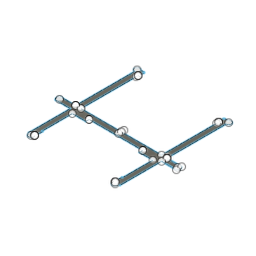
4~6F廊下用平面[少し幅大きく作ったから修正入れていこう] (Autodesk Fusion 360 design; units mm, degrees)
Autodesk Fusion 360 part; units mm, degrees
sketch "スケッチ1" plane through (0, 0, 0) normal (0, 0, 1) x (1, 0, 0)
  line L0 (-14000, -4000) -> (-54000, -4000)
  line L1 (-4000, 0) -> (-34000, 0)
  line L2 (-64000, -34500.036) -> (-64000, -33000.036)
  line L3 (-64000, -6500.036) -> (-64000, -29000.036)
  line L4 (-68000, 0) -> (-68000, 41000)
  line L5 (-54000, -6500.036) -> (-54000, -4000)
  line L6 (-64000, 0) -> (-64000, 42500)
  line L7 (-63500, 46500) -> (-64000, 46500)
  line L8 (-4000, -33000.036) -> (-4500, -33000.036)
  arc A0 (-67000, -35000) -> (-64000, -34500.036) centre (-65310.0198, -35889.9814) ccw
  line L9 (-64000, 46500) -> (-64000, 47000)
  arc A1 (11000, -4000) -> (11000, 0) centre (10000, -2000) ccw
  arc A2 (-79000, 0) -> (-79000, -4000) centre (-78000, -2000) ccw
  arc A3 (-66562.7716, 47000) -> (-68000, 43977.4822) centre (-68094.0203, 45875.1545) ccw
  line L10 (10000, 0) -> (11000, 0)
  line L11 (-64000, -33000.036) -> (-63500, -33000.036)
  line L12 (-4000, 47000) -> (-1437.2284, 47000)
  line L13 (0, 41000) -> (0, 43977.4822)
  line L14 (-4500, 42500) -> (-4500, 46500)
  line L15 (-78000, 0) -> (-79000, 0)
  line L16 (-4000, 42500) -> (-4500, 42500)
  line L17 (-4500, -29000.036) -> (-4000, -29000.036)
  line L18 (-4000, -6500.036) -> (-4000, -29000.036)
  line L19 (-64000, 42500) -> (-63500, 42500)
  line L20 (-67000, -35000) -> (-68000, -35000)
  arc A4 (-4000, -34500.036) -> (-1000, -35000) centre (-2689.9802, -35889.9814) ccw
  line L21 (-14000, -6500.036) -> (-14000, -4000)
  line L22 (-1000, -35000) -> (0, -35000)
  line L23 (-79000, -4000) -> (-68000, -4000)
  line L24 (-68000, -4000) -> (-68000, -35000)
  arc A5 (0, 43977.4822) -> (-1437.2284, 47000) centre (94.0203, 45875.1545) ccw
  line L25 (-68000, 41000) -> (-68000, 43977.4822)
  line L26 (0, 0) -> (10000, 0)
  line L27 (-68000, 0) -> (-78000, 0)
  line L28 (11000, -4000) -> (0, -4000)
  line L29 (-4500, 46500) -> (-4000, 46500)
  line L30 (-4000, 0) -> (-4000, 42500)
  line L31 (-4000, -6500.036) -> (-14000, -6500.036)
  line L32 (-4000, -34500.036) -> (-4000, -33000.036)
  line L33 (-64000, -6500.036) -> (-54000, -6500.036)
  line L34 (-4500, -33000.036) -> (-4500, -29000.036)
  line L35 (-63500, -29000.036) -> (-64000, -29000.036)
  line L36 (11000, 0) -> (0, 0)
  line L37 (-63500, -33000.036) -> (-63500, -29000.036)
  line L38 (0, 0) -> (0, 41000)
  line L39 (-34000, 2000) -> (-34000, -2000)
  line L40 (0, -4000) -> (0, -35000)
  line L41 (-64000, 47000) -> (-66562.7716, 47000)
  line L42 (-63500, 42500) -> (-63500, 46500)
  line L43 (11000, -4000) -> (0, -4000)
  line L44 (-4000, 46500) -> (-4000, 47000)
  line L45 (-64000, 0) -> (-34000, 0)
  point P0 (-4000, 0)
  point P1 (-64000, 0)
  point P2 (-4000, -35000)
  point P3 (-4000, -6500.036)
  point P4 (-64000, 41000)
  point P5 (-4000, -34500.036)
  point P6 (-4000, 42500)
  point P7 (-4000, 41000)
  point P8 (-64000, 42500)
  point P9 (-68000, 0)
  point P10 (-64000, -6500.036)
  point P11 (-64000, 0)
  point P12 (-64000, -35000)
  point P13 (-64000, -34500.036)
  constraint horizontal L0
extrude "押し出し1" add sketch "スケッチ1" along normal blind 10
